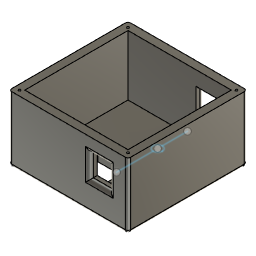
BuzzerClientTop (Autodesk Fusion 360 design; units mm, degrees)
Autodesk Fusion 360 part; units mm, degrees
sketch "Sketch13" plane through (0, 0, 0) normal (0, 0, 1) x (1, 0, 0)
  line L0 (45.45, 45.45) -> (-45.45, 45.45)
  line L1 (-45.45, 45.45) -> (-45.45, -45.45)
  line L2 (-45.45, -45.45) -> (45.45, -45.45)
  line L3 (45.45, -45.45) -> (45.45, 45.45)
  line L4 (45.45, 45.45) -> (-45.45, -45.45) construction
  line L5 (-45.45, 45.45) -> (45.45, -45.45) construction
  dimension "d87" = 90.9
  dimension "d88" = 90.9
  constraint horizontal L0
  constraint perpendicular L0 L1
  constraint parallel L0 L2
  constraint parallel L1 L3
  constraint coincident L4 origin
  constraint coincident L5 origin
  measures "d87" distance of L1.end L2.end
  measures "d88" distance of L0.end L1.end
extrude "Extrude12" add sketch "Sketch13" along normal blind 50
sketch "Sketch14" plane through (0, 0, 50) normal (0, 0, 1) x (-1, 0, 0)
  line L0 (-45.45, 45.45) -> (-45.45, -45.45)
  line L1 (-45.45, -45.45) -> (45.45, -45.45)
  line L2 (45.45, -45.45) -> (45.45, 45.45)
  line L3 (45.45, 45.45) -> (-45.45, 45.45)
  line L4 (-39.45, -39.45) -> (39.45, -39.45)
  line L5 (39.45, -39.45) -> (39.45, 39.45)
  line L6 (39.45, 39.45) -> (-39.45, 39.45)
  line L7 (-39.45, 39.45) -> (-39.45, -39.45)
  line L8 (-39.45, -39.45) -> (39.45, 39.45) construction
  line L9 (39.45, -39.45) -> (-39.45, 39.45) construction
  dimension "d91" = 78.9
  dimension "d92" = 78.9
  constraint horizontal L4
  constraint perpendicular L4 L5
  constraint parallel L4 L6
  constraint parallel L5 L7
  constraint coincident L8 origin
  constraint coincident L9 origin
  measures "d91" distance of L5.end L6.end
  measures "d92" distance of L4.end L5.end
extrude "Extrude13" cut sketch "Sketch14" against normal blind 46 contours L4 L5 L6 L7
sketch "Sketch15" plane through (0, 0, 50) normal (0, 0, 1) x (-1, 0, 0)
  line L0 (39.45, -39.45) -> (-39.45, -39.45)
  line L1 (-39.45, -39.45) -> (-39.45, 39.45)
  line L2 (-39.45, 39.45) -> (39.45, 39.45)
  line L3 (39.45, 39.45) -> (39.45, -39.45)
  line L4 (-45.45, 45.45) -> (-45.45, -45.45)
  line L5 (-45.45, -45.45) -> (45.45, -45.45)
  line L6 (45.45, -45.45) -> (45.45, 45.45)
  line L7 (45.45, 45.45) -> (-45.45, 45.45)
  line L8 (45.45, -45.45) -> (41.45, -45.45)
  line L9 (45.45, -41.45) -> (45.45, -45.45)
  circle A0 centre (41.45, -41.45) radius 0.85
  line L10 (-45.45, -45.45) -> (-41.45, -45.45)
  line L11 (-45.45, -41.45) -> (-45.45, -45.45)
  circle A1 centre (-41.45, -41.45) radius 0.85
  line L12 (45.45, 45.45) -> (41.45, 45.45)
  line L13 (41.45, 45.45) -> (41.45, 42.3)
  line L14 (45.45, 41.45) -> (45.45, 45.45)
  circle A2 centre (41.45, 41.45) radius 0.85
  line L15 (-45.45, 45.45) -> (-41.45, 45.45)
  line L16 (-45.45, 41.45) -> (-45.45, 45.45)
  circle A3 centre (-41.45, 41.45) radius 0.85
  line L17 (-41.45, 45.45) -> (-41.45, 42.3)
  line L18 (-42.3, 41.45) -> (-45.45, 41.45)
  line L19 (42.3, 41.45) -> (45.45, 41.45)
  line L20 (41.45, -45.45) -> (41.45, -42.3)
  line L21 (42.3, -41.45) -> (45.45, -41.45)
  line L22 (-41.45, -45.45) -> (-41.45, -42.3)
  line L23 (-42.3, -41.45) -> (-45.45, -41.45)
  dimension "d95" = 4
  dimension "d96" = 4
  dimension "d97" = 1.7
  dimension "d98" = 4
  dimension "d99" = 4
  dimension "d100" = 1.7
  dimension "d101" = 4
  dimension "d102" = 4
  dimension "d103" = 1.7
  dimension "d104" = 4
  dimension "d105" = 4
  dimension "d106" = 1.7
  constraint horizontal L8
  constraint vertical L9
  constraint coincident L5.end L6.start
  constraint horizontal L10
  constraint vertical L11
  constraint coincident L4.end L5.start
  constraint horizontal L12
  constraint vertical L13
  constraint vertical L14
  constraint coincident L6.end L7.start
  constraint horizontal L15
  constraint vertical L16
  constraint coincident L4.start L7.end
  constraint coincident A3 L17.end
  constraint vertical L17
  constraint coincident A3 L18.start
  constraint horizontal L18
  constraint coincident A2 L19.start
  constraint horizontal L19
  constraint coincident A2 L13.end
  constraint coincident A0 L20.end
  constraint vertical L20
  constraint coincident A0 L21.start
  constraint horizontal L21
  constraint coincident A1 L22.end
  constraint vertical L22
  constraint coincident A1 L23.start
  constraint horizontal L23
  measures "d95" distance of L5.end L8.end
  measures "d96" distance of L5.end L9.start
  measures "d97" diameter of A0
  measures "d98" distance of L4.end L10.end
  measures "d99" distance of L4.end L11.start
  measures "d100" diameter of A1
  measures "d101" distance of L6.end L12.end
  measures "d102" distance of L6.end L14.start
  measures "d103" diameter of A2
  measures "d104" distance of L4.start L15.end
  measures "d105" distance of L4.start L16.start
  measures "d106" diameter of A3
extrude "Extrude14" cut sketch "Sketch15" against normal blind 20 contours A3 | A1 | A2 | A0
sketch "Sketch16" plane through (0, 0, 0) normal (0, 0, 1) x (1, 0, 0)
  circle A0 centre (0, 22.6858) radius 3.5
  line L0 (0, 45.4608) -> (0, 26.1858)
  line L1 (0, 19.1858) -> (0, -8.7142)
  dimension "d109" = 22.775
  dimension "d110" = 7
  constraint coincident A0 L0.end
  constraint vertical L0
  constraint vertical L1
  constraint coincident A0 L1.start
  measures "d109" distance of L0.start A0.centre
  measures "d110" diameter of A0
extrude "Extrude15" cut sketch "Sketch16" along normal blind 4
sketch "Sketch17" plane through (0, -39.45, 0) normal (0, 1, 0) x (-1, 0, 0)
  line L0 (39.45, 50) -> (-39.45, 50)
  line L1 (-39.45, 50) -> (-39.45, 4)
  line L2 (-39.45, 4) -> (39.45, 4)
  line L3 (39.45, 4) -> (39.45, 50)
  line L4 (-39.45, 50) -> (-32.355, 50)
  line L5 (-32.355, 50) -> (-32.355, 39)
  line L6 (-32.355, 39) -> (-39.45, 39)
  line L7 (-39.45, 39) -> (-39.45, 50)
  line L8 (-32.355, 39) -> (-31.155, 39)
  line L9 (-31.155, 39) -> (-15.955, 39)
  line L10 (-15.955, 39) -> (-15.955, 23.176)
  line L11 (-31.155, 21) -> (-31.155, 39)
  line L12 (-31.155, 24.4) -> (-31.155, 21.176)
  line L13 (-31.155, 21.176) -> (-15.955, 21.176)
  line L14 (-15.955, 21.176) -> (-15.955, 23.176)
  dimension "d113" = 7.095
  dimension "d114" = 11
  dimension "d115" = 1.2
  dimension "d116" = 15.2
  dimension "d117" = 18
  dimension "d248" = 2
  constraint horizontal L4
  constraint vertical L5
  constraint horizontal L6
  constraint vertical L7
  constraint coincident L0.end L1.start
  constraint perpendicular L5 L8
  constraint horizontal L9
  constraint vertical L10
  constraint vertical L11
  constraint vertical L12
  constraint horizontal L13
  constraint vertical L14
  measures "d113" distance of L0.end L4.end
  measures "d114" distance of L0.end L6.end
  measures "d115" distance of L5.end L8.end
  measures "d116" distance of L8.end L9.end
  measures "d117" distance of L8.end L11.start
  measures "d248" distance of L10.end L13.end
extrude "Extrude16" cut sketch "Sketch17" against normal blind 10 contours L9 L10 L11 L12 L13 L14
sketch "Sketch18" plane through (0, 39.45, 0) normal (0, -1, 0) x (1, 0, 0)
  line L0 (39.45, 50) -> (-39.45, 50)
  line L1 (-39.45, 50) -> (-39.45, 4)
  line L2 (-39.45, 4) -> (39.45, 4)
  line L3 (39.45, 4) -> (39.45, 50)
  line L4 (39.45, 50) -> (28.92, 50)
  line L5 (28.92, 50) -> (28.92, 39)
  line L6 (28.92, 39) -> (39.45, 39)
  line L7 (39.45, 39) -> (39.45, 50)
  line L8 (28.92, 39) -> (27.72, 39)
  line L9 (27.72, 39) -> (12.52, 39)
  line L10 (12.52, 39) -> (12.52, 22.7867)
  line L11 (27.72, 21) -> (27.72, 39)
  line L12 (27.72, 24.4) -> (27.72, 20.7867)
  line L13 (27.72, 20.7867) -> (12.52, 20.7867)
  line L14 (12.52, 20.7867) -> (12.52, 22.7867)
  dimension "d120" = 10.53
  dimension "d121" = 11
  dimension "d122" = 1.2
  dimension "d123" = 15.2
  dimension "d124" = 18
  dimension "d249" = 2
  constraint horizontal L4
  constraint vertical L5
  constraint horizontal L6
  constraint vertical L7
  constraint coincident L0.start L3.end
  constraint perpendicular L5 L8
  constraint horizontal L9
  constraint vertical L10
  constraint vertical L11
  constraint vertical L12
  constraint horizontal L13
  constraint vertical L14
  measures "d120" distance of L0.start L4.end
  measures "d121" distance of L0.start L6.end
  measures "d122" distance of L5.end L8.end
  measures "d123" distance of L8.end L9.end
  measures "d124" distance of L8.end L11.start
  measures "d249" distance of L10.end L13.end
extrude "Extrude17" cut sketch "Sketch18" against normal blind 10 contours L9 L10 L11 L12 L13 L14
fillet "Fillet1" radius 2 8 edges at (45.45, -45.45, 25) (45.45, 0, 0) (0, -45.45, 0) (-45.45, -45.45, 25) (45.45, 45.45, 25) (-45.45, 45.45, 25) (-45.45, 0, 0) (0, 45.45, 0)
fillet "Fillet8" radius 3 4 edges at (12.52, 45.45, 29.8934) (20.12, 45.45, 39) (27.72, 45.45, 29.8934) (20.12, 45.45, 20.7867)
fillet "Fillet9" radius 3 4 edges at (31.155, -45.45, 30.088) (23.555, -45.45, 39) (15.955, -45.45, 30.088) (23.555, -45.45, 21.176)
thread "Thread5" "ISO Metric profile 7.0 M7x0.5 6H" major diameter 7.0922 minor diameter 6.5287 pitch 0.5 angle 60 modelled right hand crest width 0.133 on face at (3.4826, 22.3373, 1.3333) crest through (3.2644, 22.6858, 0.125)
sketch "Sketch27" plane through (0, 0, 4) normal (0, 0, 1) x (-1, 0, 0)
  line L0 (-39.45, 39.45) -> (-39.45, -39.45)
  line L1 (-39.45, -39.45) -> (39.45, -39.45)
  line L2 (39.45, -39.45) -> (39.45, 39.45)
  line L3 (39.45, 39.45) -> (-39.45, 39.45)
  line L4 (16, 4.475) -> (-16, 4.475)
  line L5 (-16, 4.475) -> (-16, 34.475)
  line L6 (-16, 34.475) -> (16, 34.475)
  line L7 (16, 34.475) -> (16, 4.475)
  line L8 (16, 4.475) -> (-16, 34.475) construction
  line L9 (-16, 4.475) -> (16, 34.475) construction
  line L10 (14, 29.975) -> (-14, 29.975)
  line L11 (-14, 29.975) -> (-14, 8.975)
  line L12 (-14, 8.975) -> (14, 8.975)
  line L13 (14, 8.975) -> (14, 29.975)
  line L14 (14, 29.975) -> (-14, 8.975) construction
  line L15 (-14, 29.975) -> (14, 8.975) construction
  spline S0 degree 3 poles (-0.9171, -26.1112) (-1.3546, -25.9757) (-1.7616, -25.7566) (-2.4627, -25.1781) (-2.7516, -24.8264) (-3.174, -24.0374) (-3.3057, -23.609) (-3.3954, -22.7326) (-3.3553, -22.2933) (-3.1547, -21.6147) (-3.0466, -21.3654) (-2.7732, -20.9013) (-2.6096, -20.6879) (-2.4217, -20.4968) knots 0 0 0 0 0.137406 0.137406 0.27276 0.27276 0.406063 0.406063 0.537313 0.537313 0.618635 0.618635 0.69914 0.69914 0.69914 0.69914
  arc A0 (2.4217, -20.4968) -> (-2.4217, -20.4968) centre (0, -22.6858) ccw
  spline S1 degree 3 poles (2.4217, -20.4968) (2.7219, -20.802) (2.9591, -21.1634) (3.2856, -21.9626) (3.3692, -22.3938) (3.3677, -23.2712) (3.28, -23.7088) (2.9403, -24.5328) (2.6891, -24.9102) (2.1721, -25.4323) (1.947, -25.6096) (1.4564, -25.9073) (1.1925, -26.0259) (0.9171, -26.1112) knots 0 0 0 0 0.128434 0.128434 0.258917 0.258917 0.391449 0.391449 0.52603 0.52603 0.61157 0.61157 0.697927 0.697927 0.697927 0.697927
  arc A1 (-0.9171, -26.1112) -> (0.9171, -26.1112) centre (0, -22.6858) ccw
  point P0 (0, 19.475)
  point P1 (0, 19.475)
  dimension "d274" = 32
  dimension "d275" = 30
  dimension "d276" = 28
  dimension "d277" = 21
  constraint horizontal L4
  constraint perpendicular L4 L5
  constraint parallel L4 L6
  constraint parallel L5 L7
  constraint coincident L8 P1
  constraint coincident L9 P1
  constraint horizontal L10
  constraint perpendicular L10 L11
  constraint parallel L10 L12
  constraint parallel L11 L13
  constraint coincident L14 P1
  constraint coincident L15 P1
  constraint coincident P1 P0
  measures "d274" distance of L5.end L6.end
  measures "d275" distance of L4.end L5.end
  measures "d276" distance of L11.end L12.end
  measures "d277" distance of L10.end L11.end
extrude "Extrude35" add sketch "Sketch27" along normal blind 7 contours L4 L5 L6 L7
sketch "Sketch28" plane through (0, 0, 11) normal (0, 0, 1) x (-1, 0, 0)
  line L0 (14, 29.975) -> (14, 8.975)
  line L1 (14, 8.975) -> (-14, 8.975)
  line L2 (-14, 8.975) -> (-14, 29.975)
  line L3 (-14, 29.975) -> (14, 29.975)
  line L4 (16, 34.475) -> (-16, 34.475)
  line L5 (-16, 34.475) -> (-16, 4.475)
  line L6 (-16, 4.475) -> (16, 4.475)
  line L7 (16, 4.475) -> (16, 34.475)
  line L8 (-7, 34.475) -> (7, 34.475)
  line L9 (7, 34.475) -> (7, 30.775)
  line L10 (7, 30.775) -> (-7, 30.775)
  line L11 (-7, 30.775) -> (-7, 34.475)
  dimension "d280" = 14
  dimension "d281" = 3.7
  constraint horizontal L8
  constraint vertical L9
  constraint horizontal L10
  constraint vertical L11
  constraint coincident L4 L8.start
  constraint midpoint L4 L8
  measures "d280" distance of L8.start L8.end
  measures "d281" distance of L8.start L10.end
extrude "Extrude36" cut sketch "Sketch28" against normal blind 3 contours L4 L8 L9 L10 L11
sketch "Sketch29" plane through (0, 0, 11) normal (0, 0, 1) x (-1, 0, 0)
  line L0 (-7, 30.775) -> (-7, 34.475)
  line L1 (-7, 34.475) -> (-16, 34.475)
  line L2 (-16, 34.475) -> (-16, 4.475)
  line L3 (-16, 4.475) -> (16, 4.475)
  line L4 (16, 4.475) -> (16, 34.475)
  line L5 (16, 34.475) -> (7, 34.475)
  line L6 (7, 34.475) -> (7, 30.775)
  line L7 (7, 30.775) -> (-7, 30.775)
  line L8 (14, 29.975) -> (14, 8.975)
  line L9 (14, 8.975) -> (-14, 8.975)
  line L10 (-14, 8.975) -> (-14, 29.975)
  line L11 (-14, 29.975) -> (14, 29.975)
  line L12 (13.3, 33.475) -> (-14.2, 33.475)
  line L13 (-14.2, 33.475) -> (-14.2, 5.975)
  line L14 (-14.2, 5.975) -> (13.3, 5.975)
  line L15 (13.3, 5.975) -> (13.3, 33.475)
  line L16 (13.3, 33.475) -> (-14.2, 5.975) construction
  line L17 (-14.2, 33.475) -> (13.3, 5.975) construction
  line L18 (-14.2, 33.475) -> (-12.7, 33.475)
  line L19 (-14.2, 31.975) -> (-14.2, 33.475)
  line L20 (13.3, 33.475) -> (11.8, 33.475)
  line L21 (13.3, 31.975) -> (13.3, 33.475)
  line L22 (-14.2, 5.975) -> (-12.7, 5.975)
  line L23 (-11.7, 7.475) -> (-14.2, 7.475)
  line L24 (-14.2, 7.475) -> (-14.2, 5.975)
  line L25 (13.3, 5.975) -> (11.8, 5.975)
  line L26 (13.3, 7.475) -> (13.3, 5.975)
  circle A0 centre (-11.7, 30.975) radius 0.85
  circle A1 centre (11.8, 30.975) radius 0.85
  circle A2 centre (-11.7, 7.475) radius 0.85
  circle A3 centre (11.8, 7.475) radius 0.85
  line L27 (14, 29.975) -> (11.8, 29.975)
  line L28 (14, 30.975) -> (14, 29.975)
  line L29 (11.8, 30.975) -> (-11.7, 30.975)
  line L30 (11.8, 30.975) -> (11.8, 7.475)
  line L31 (-11.7, 30.975) -> (-11.7, 7.475)
  point P0 (-0.45, 19.725)
  dimension "d284" = 27.5
  dimension "d285" = 27.5
  dimension "d286" = 1.5
  dimension "d287" = 1.5
  dimension "d288" = 1.5
  dimension "d289" = 1.5
  dimension "d290" = 1.5
  dimension "d291" = 1.5
  dimension "d292" = 1.5
  dimension "d293" = 1.5
  dimension "d294" = 1.7
  dimension "d295" = 1.7
  dimension "d296" = 1.7
  dimension "d297" = 1.7
  dimension "d302" = 2.2
  dimension "d303" = 1
  dimension "d304" = 23.5
  dimension "d305" = 23.5
  dimension "d306" = 23.5
  constraint horizontal L12
  constraint perpendicular L12 L13
  constraint parallel L12 L14
  constraint parallel L13 L15
  constraint coincident L16 P0
  constraint coincident L17 P0
  constraint horizontal L18
  constraint vertical L19
  constraint horizontal L20
  constraint vertical L21
  constraint horizontal L22
  constraint horizontal L23
  constraint vertical L24
  constraint horizontal L25
  constraint vertical L26
  constraint coincident L23.start A2.centre
  constraint horizontal L27
  constraint vertical L28
  constraint coincident L8.start L11.end
  constraint coincident A1.centre L29.start
  constraint perpendicular L8 L29
  constraint coincident A0.centre L29.end
  constraint perpendicular L29 L30
  constraint perpendicular L29 L31
  constraint coincident A3.centre L30.end
  measures "d284" distance of L13.end L14.end
  measures "d285" distance of L12.end L13.end
  measures "d286" distance of L12.end L18.end
  measures "d287" distance of L12.end L19.start
  measures "d288" distance of L12.start L20.end
  measures "d289" distance of L12.start L21.start
  measures "d290" distance of L13.end L22.end
  measures "d291" distance of L13.end L23.end
  measures "d292" distance of L14.end L25.end
  measures "d293" distance of L14.end L26.start
  measures "d294" diameter of A0
  measures "d295" diameter of A1
  measures "d296" diameter of A2
  measures "d297" diameter of A3
  measures "d302" distance of L8.start L27.end
  measures "d303" distance of L8.start L28.start
  measures "d304" distance of A1.centre A0.centre
  measures "d305" distance of A1.centre A3.centre
  measures "d306" distance of A0.centre L23.start
extrude "Extrude37" cut sketch "Sketch29" against normal blind 9 contours A0 L29 L31 | A0 L29 L31 | A1 L29 L30 | A1 L29 L30 | L23 A2 L31 | L23 A2 L31 | A3
extrude "Extrude38" cut 1 faces at (4.6667, -15.975, 4) along direction (0, 0, -1) blind 5
